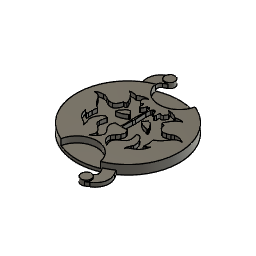
Deckbox - Key - Rakdos (Autodesk Fusion 360 design; units mm, degrees)
Autodesk Fusion 360 part; units mm, degrees
sketch "Sketch1" plane through (0, 0, 0) normal (0, 1, 0) x (1, 0, 0)
  circle A0 centre (0, 0) radius 25.4
  line L0 (19.5918, -28.934) -> (-15.2617, 31.434)
  line L1 (-19.5918, 28.934) -> (15.2617, -31.434)
  line L2 (0, -25.4) -> (0, 25.4) construction
  line L3 (0, 0) -> (25.4, 0) construction
  line L4 (-19.5918, 28.934) -> (-15.2617, 31.434)
  line L5 (15.2617, -31.434) -> (19.5918, -28.934)
  line L6 (17.4268, -30.184) -> (-17.4268, 30.184) construction
  line L7 (-2.1651, -1.25) -> (2.1651, 1.25) construction
  line L8 (19.5918, -28.934) -> (11.7976, -33.434)
  line L9 (11.7976, -33.434) -> (9.2976, -29.1039)
  line L10 (9.2976, -29.1039) -> (17.0918, -24.6039)
  line L11 (17.0918, -24.6039) -> (19.5918, -28.934)
  circle A1 centre (10.5476, -31.269) radius 2.5
  circle A2 centre (0, 0) radius 35.5
  line L12 (-19.5918, 28.934) -> (-17.0918, 24.6039)
  line L13 (-17.0918, 24.6039) -> (-9.2976, 29.1039)
  line L14 (-9.2976, 29.1039) -> (-11.7976, 33.434)
  line L15 (-11.7976, 33.434) -> (-19.5918, 28.934)
  circle A3 centre (-10.5476, 31.269) radius 2.5
  point P0 (-12.5, 21.6506)
  point P1 (12.5, -21.6506)
  dimension "d1" = 50.8
  dimension "d42" = 5
  dimension "d45" = 5
  dimension "d46" = 71
  dimension "d47" = 60
  dimension "d48" = 4
  dimension "d51" = 5
  constraint coincident A0.centre L3.start
  constraint coincident A0 L2.start
  constraint coincident A0 L2.end
  constraint coincident A0.centre L2
  constraint coincident A0 L3.end
  constraint horizontal L3
  constraint perpendicular L0 L4
  constraint perpendicular L0 L5
  constraint perpendicular L1 L4
  constraint midpoint L5 L6.start
  constraint midpoint L4 L6.end
  constraint perpendicular L4 L6
  constraint midpoint L1 L7.start
  constraint midpoint L0 L7.end
  constraint midpoint L6 A0.centre
  constraint perpendicular L8 L9
  constraint parallel L8 L10
  constraint parallel L9 L11
  constraint perpendicular L0 L8
  constraint midpoint L9 A1.centre
  constraint tangent L10 A1
  constraint concentric A0 A2
  constraint tangent A1 A2
  constraint perpendicular L12 L13
  constraint parallel L12 L14
  constraint parallel L13 L15
  constraint coincident L1 L12.end
  constraint midpoint L14 A3.centre
  constraint tangent L13 A3
  constraint tangent A2 A3
  measures "d1" diameter of A0
  measures "d42" distance of L0 L1
  measures "d45" diameter of A1
  measures "d46" diameter of A2 A0.centre
  measures "d47" angle of L3 L6
  measures "d48" distance of L1 A1.centre
  measures "d51" diameter of A3
extrude "Extrude1" add sketch "Sketch1" along normal blind 4.5 contours A0 L0 | A0 L0 L1 | A0 L1
extrude "Extrude2" add sketch "Sketch1" along normal blind 1.9 contours A0 L0 | A0 L0 L1 | A0 L0 L1 L13 | A0 L0 L1 L10 | A0 L1 | L0 L1 L4 L12 L13 L15 | L0 L13 L15 A3 | L0 L1 L5 L8 L10 L11 | L14 A3 | L14 A3 | L1 L8 L10 A1 | L9 A1 | L9 A1
extrude "Extrude3" add sketch "Sketch1" along normal blind 2.5 contours L14 A3 | L14 A3 | L9 A1 | L9 A1
sketch "Sketch2" plane through (0, 4.5, 0) normal (0, 1, 0) x (-1, 0, 0)
  circle A0 centre (0, 0) radius 25.4
  circle A1 centre (0, -25.4) radius 10
  circle A2 centre (0, 25.4) radius 10
  line L0 (0, -25.4) -> (0, 25.4) construction
  dimension "d18" = 20
  dimension "d19" = 20
  constraint coincident A0 A1.centre
  constraint coincident A0 A2.centre
  constraint coincident A1.centre L0.start
  constraint coincident A2.centre L0.end
  constraint coincident A0.centre L0
  constraint vertical L0
  measures "d18" diameter of A1
  measures "d19" diameter of A2
extrude "Extrude4" cut sketch "Sketch2" against normal blind 3 contours A0 A2 | A0 A1 picked at (-1.832, 22.0709) picked at (1.832, -22.0709)
fillet "Fillet6" radius 2 2 edges at (12.7617, 0.95, 27.1039) (-12.7617, 0.95, -27.1039)
fillet "Fillet7" radius 7 2 edges at (19.5918, 0.95, 28.934) (-19.5918, 0.95, -28.934)
sketch "Sketch3" plane through (0, 4.5, 0) normal (0, 1, 0) x (-1, 0, 0)
  arc A0 (-9.8043, 23.4315) -> (-9.8043, -23.4315) centre (0, 0) ccw
  spline S0 degree 3 poles (-4.3232, 14.8555) (-4.3232, 14.84) (-4.2479, 14.6896) (-4.114, 14.4374) knots 0 0 0 0 1 1 1 1
  spline S1 degree 3 poles (-4.114, 14.4374) (-3.4685, 13.2223) (-3.3365, 12.5312) (-3.5867, 11.6779) knots 0 0 0 0 1 1 1 1
  spline S2 degree 3 poles (-3.5867, 11.6779) (-3.8334, 10.8365) (-4.2867, 10.3197) (-5.7211, 9.2444) knots 0 0 0 0 1 1 1 1
  spline S3 degree 3 poles (-5.7211, 9.2444) (-6.746, 8.4761) (-7.0061, 8.2496) (-7.3329, 7.8412) knots 0 0 0 0 1 1 1 1
  spline S4 degree 3 poles (-7.3329, 7.8412) (-7.7451, 7.3262) (-7.9627, 6.6689) (-7.8957, 6.1401) knots 0 0 0 0 1 1 1 1
  spline S5 degree 3 poles (-7.8957, 6.1401) (-7.8192, 5.5352) (-7.453, 3.8698) (-7.2145, 3.0422) knots 0 0 0 0 1 1 1 1
  spline S6 degree 3 poles (-7.2145, 3.0422) (-7.1781, 2.9158) (-7.1519, 2.8094) (-7.1563, 2.8056) knots 0 0 0 0 1 1 1 1
  spline S7 degree 3 poles (-7.1563, 2.8056) (-7.1605, 2.8018) (-7.2159, 2.7934) (-7.2792, 2.7869) knots 0 0 0 0 1 1 1 1
  spline S8 degree 3 poles (-7.2792, 2.7869) (-7.4349, 2.771) (-7.9577, 2.711) (-8.2149, 2.6796) knots 0 0 0 0 1 1 1 1
  line L0 (-8.2149, 2.6796) -> (-8.424, 2.6541)
  line L1 (-8.424, 2.6541) -> (-8.5105, 2.7114)
  spline S9 degree 3 poles (-8.5105, 2.7114) (-9.2284, 3.1878) (-9.9979, 4.0729) (-10.5135, 5.0154) knots 0 0 0 0 1 1 1 1
  spline S10 degree 3 poles (-10.5135, 5.0154) (-11.1798, 6.2335) (-11.3977, 7.5273) (-11.0924, 8.4525) knots 0 0 0 0 1 1 1 1
  spline S11 degree 3 poles (-11.0924, 8.4525) (-11.0292, 8.6439) (-10.9777, 8.7574) (-10.7473, 9.2134) knots 0 0 0 0 1 1 1 1
  spline S12 degree 3 poles (-10.7473, 9.2134) (-10.4288, 9.844) (-10.3072, 10.1818) (-10.2108, 10.705) knots 0 0 0 0 1 1 1 1
  spline S13 degree 3 poles (-10.2108, 10.705) (-10.1491, 11.0402) (-10.0941, 11.5884) (-10.0956, 11.8545) knots 0 0 0 0 1 1 1 1
  line L2 (-10.0956, 11.8545) -> (-10.096, 11.9297)
  line L3 (-10.096, 11.9297) -> (-10.135, 11.8125)
  spline S14 degree 3 poles (-10.135, 11.8125) (-10.3374, 11.2033) (-10.7118, 10.8714) (-11.9958, 10.1624) knots 0 0 0 0 1 1 1 1
  spline S15 degree 3 poles (-11.9958, 10.1624) (-12.7961, 9.7205) (-13.1607, 9.495) (-13.5622, 9.1932) knots 0 0 0 0 1 1 1 1
  spline S16 degree 3 poles (-13.5622, 9.1932) (-14.8947, 8.1916) (-15.6884, 6.8114) (-16.0072, 4.9415) knots 0 0 0 0 1 1 1 1
  spline S17 degree 3 poles (-16.0072, 4.9415) (-16.0323, 4.794) (-16.0296, 4.7863) (-15.9839, 4.8766) knots 0 0 0 0 1 1 1 1
  spline S18 degree 3 poles (-15.9839, 4.8766) (-15.749, 5.3417) (-15.2485, 5.7388) (-14.8855, 5.7479) knots 0 0 0 0 1 1 1 1
  line L4 (-14.8855, 5.7479) -> (-14.7907, 5.7503)
  line L5 (-14.7907, 5.7503) -> (-14.7317, 5.8382)
  spline S19 degree 3 poles (-14.7317, 5.8382) (-14.4686, 6.2307) (-14.147, 6.5223) (-13.9762, 6.5233) knots 0 0 0 0 1 1 1 1
  spline S20 degree 3 poles (-13.9762, 6.5233) (-13.9206, 6.5236) (-13.9207, 6.5239) (-13.9435, 6.3922) knots 0 0 0 0 1 1 1 1
  spline S21 degree 3 poles (-13.9435, 6.3922) (-13.9836, 6.1605) (-14.019, 5.8212) (-14.0453, 5.4163) knots 0 0 0 0 1 1 1 1
  spline S22 degree 3 poles (-14.0453, 5.4163) (-14.0629, 5.1457) (-14.063, 3.8981) (-14.0455, 3.6225) knots 0 0 0 0 1 1 1 1
  spline S23 degree 3 poles (-14.0455, 3.6225) (-13.9774, 2.5472) (-13.8599, 1.834) (-13.6638, 1.3035) knots 0 0 0 0 1 1 1 1
  spline S24 degree 3 poles (-13.6638, 1.3035) (-13.6467, 1.2571) (-13.6336, 1.2182) (-13.635, 1.217) knots 0 0 0 0 1 1 1 1
  spline S25 degree 3 poles (-13.635, 1.217) (-13.6363, 1.2158) (-13.6892, 1.1889) (-13.7527, 1.1573) knots 0 0 0 0 1 1 1 1
  spline S26 degree 3 poles (-13.7527, 1.1573) (-14.5202, 0.7741) (-15.2509, 0.2522) (-15.8555, -0.3449) knots 0 0 0 0 1 1 1 1
  spline S27 degree 3 poles (-15.8555, -0.3449) (-16.4345, -0.9167) (-16.8065, -1.4006) (-17.5005, -2.4852) knots 0 0 0 0 1 1 1 1
  spline S28 degree 3 poles (-17.5005, -2.4852) (-18.1246, -3.4604) (-18.4276, -3.851) (-18.8281, -4.1974) knots 0 0 0 0 1 1 1 1
  spline S29 degree 3 poles (-18.8281, -4.1974) (-19.5229, -4.798) (-20.2555, -5.0448) (-21.5036, -5.0986) knots 0 0 0 0 1 1 1 1
  line L6 (-21.5036, -5.0986) -> (-21.664, -5.1056)
  line L7 (-21.664, -5.1056) -> (-21.6039, -5.1535)
  spline S30 degree 3 poles (-21.6039, -5.1535) (-21.2674, -5.4216) (-20.7454, -5.6937) (-20.2337, -5.8676) knots 0 0 0 0 1 1 1 1
  spline S31 degree 3 poles (-20.2337, -5.8676) (-19.1845, -6.2243) (-17.7553, -6.3205) (-16.9672, -6.0873) knots 0 0 0 0 1 1 1 1
  spline S32 degree 3 poles (-16.9672, -6.0873) (-16.6077, -5.9811) (-16.3618, -5.8552) (-15.8069, -5.4933) knots 0 0 0 0 1 1 1 1
  spline S33 degree 3 poles (-15.8069, -5.4933) (-15.0981, -5.0312) (-14.8175, -4.8913) (-14.3139, -4.7489) knots 0 0 0 0 1 1 1 1
  spline S34 degree 3 poles (-14.3139, -4.7489) (-13.6862, -4.5713) (-12.7854, -4.5135) (-12.307, -4.6201) knots 0 0 0 0 1 1 1 1
  spline S35 degree 3 poles (-12.307, -4.6201) (-11.2155, -4.8633) (-10.4225, -5.9028) (-9.9684, -7.6859) knots 0 0 0 0 1 1 1 1
  spline S36 degree 3 poles (-9.9684, -7.6859) (-9.9326, -7.8264) (-9.899, -7.9583) (-9.8937, -7.9789) knots 0 0 0 0 1 1 1 1
  line L8 (-9.8937, -7.9789) -> (-9.8839, -8.0165)
  line L9 (-9.8839, -8.0165) -> (-9.8344, -7.9914)
  spline S37 degree 3 poles (-9.8344, -7.9914) (-9.4661, -7.8047) (-9.0003, -7.8234) (-8.7851, -8.0334) knots 0 0 0 0 1 1 1 1
  spline S38 degree 3 poles (-8.7851, -8.0334) (-8.5675, -8.2459) (-8.6314, -8.5665) (-9.0766, -9.4946) knots 0 0 0 0 1 1 1 1
  spline S39 degree 3 poles (-9.0766, -9.4946) (-10.0976, -11.6236) (-11.5586, -13.2241) (-13.0137, -13.8076) knots 0 0 0 0 1 1 1 1
  spline S40 degree 3 poles (-13.0137, -13.8076) (-13.1416, -13.8589) (-13.1411, -13.8575) (-13.0478, -13.8967) knots 0 0 0 0 1 1 1 1
  spline S41 degree 3 poles (-13.0478, -13.8967) (-12.3642, -14.1837) (-10.9358, -14.1235) (-9.6156, -13.7521) knots 0 0 0 0 1 1 1 1
  line L10 (-9.6156, -13.7521) -> (-9.492, -13.7173)
  line L11 (-9.492, -13.7173) -> (-9.4096, -13.7964)
  spline S42 degree 3 poles (-9.4096, -13.7964) (-8.7246, -14.4541) (-7.3203, -15.0258) (-6.0462, -15.1659) knots 0 0 0 0 1 1 1 1
  spline S43 degree 3 poles (-6.0462, -15.1659) (-5.675, -15.2066) (-4.8009, -15.2092) (-4.9044, -15.1692) knots 0 0 0 0 1 1 1 1
  spline S44 degree 3 poles (-4.9044, -15.1692) (-4.9126, -15.1661) (-4.9487, -15.1535) (-4.9846, -15.1412) knots 0 0 0 0 1 1 1 1
  spline S45 degree 3 poles (-4.9846, -15.1412) (-5.6774, -14.9038) (-6.4552, -14.0325) (-6.46, -13.4885) knots 0 0 0 0 1 1 1 1
  spline S46 degree 3 poles (-6.46, -13.4885) (-6.4631, -13.1388) (-6.0298, -12.3937) (-5.5419, -11.9095) knots 0 0 0 0 1 1 1 1
  spline S47 degree 3 poles (-5.5419, -11.9095) (-4.927, -11.2995) (-4.4549, -11.3506) (-4.2518, -12.0497) knots 0 0 0 0 1 1 1 1
  spline S48 degree 3 poles (-4.2518, -12.0497) (-4.2241, -12.1449) (-4.2303, -12.1478) (-4.1399, -11.9973) knots 0 0 0 0 1 1 1 1
  spline S49 degree 3 poles (-4.1399, -11.9973) (-3.7726, -11.3854) (-3.7203, -10.8265) (-3.9765, -10.2475) knots 0 0 0 0 1 1 1 1
  line L12 (-3.9765, -10.2475) -> (-4.0011, -10.1919)
  line L13 (-4.0011, -10.1919) -> (-3.9349, -10.0737)
  spline S50 degree 3 poles (-3.9349, -10.0737) (-3.8628, -9.9448) (-3.7451, -9.7037) (-3.662, -9.5147) knots 0 0 0 0 1 1 1 1
  spline S51 degree 3 poles (-3.662, -9.5147) (-3.6329, -9.4485) (-3.603, -9.3823) (-3.5955, -9.3676) knots 0 0 0 0 1 1 1 1
  line L14 (-3.5955, -9.3676) -> (-3.5818, -9.3406)
  line L15 (-3.5818, -9.3406) -> (-3.5191, -9.3586)
  spline S52 degree 3 poles (-3.5191, -9.3586) (-2.8503, -9.5507) (-2.4025, -10.1704) (-2.0524, -11.3885) knots 0 0 0 0 1 1 1 1
  spline S53 degree 3 poles (-2.0524, -11.3885) (-1.9105, -11.882) (-1.9247, -11.86) (-1.8216, -11.7507) knots 0 0 0 0 1 1 1 1
  spline S54 degree 3 poles (-1.8216, -11.7507) (-1.5685, -11.4824) (-1.3668, -11.0199) (-1.4199, -10.8299) knots 0 0 0 0 1 1 1 1
  spline S55 degree 3 poles (-1.4199, -10.8299) (-1.4388, -10.7621) (-1.2673, -10.8106) (-1.1899, -10.895) knots 0 0 0 0 1 1 1 1
  spline S56 degree 3 poles (-1.1899, -10.895) (-1.0195, -11.0806) (-1.0394, -11.4423) (-1.2358, -11.7278) knots 0 0 0 0 1 1 1 1
  spline S57 degree 3 poles (-1.2358, -11.7278) (-1.2529, -11.7526) (-1.2669, -11.7771) (-1.2669, -11.7822) knots 0 0 0 0 1 1 1 1
  spline S58 degree 3 poles (-1.2669, -11.7822) (-1.2669, -11.8057) (-0.9842, -11.8254) (-0.8973, -11.8081) knots 0 0 0 0 1 1 1 1
  spline S59 degree 3 poles (-0.8973, -11.8081) (-0.8351, -11.7957) (-0.5203, -11.2526) (-0.3903, -10.9336) knots 0 0 0 0 1 1 1 1
  spline S60 degree 3 poles (-0.3903, -10.9336) (-0.1766, -10.4095) (-0.1031, -9.7731) (-0.1337, -8.7129) knots 0 0 0 0 1 1 1 1
  spline S61 degree 3 poles (-0.1337, -8.7129) (-0.1691, -7.4849) (-0.2863, -4.5446) (-0.3463, -3.3794) knots 0 0 0 0 1 1 1 1
  spline S62 degree 3 poles (-0.3463, -3.3794) (-0.36, -3.1128) (-0.3567, -3.0373) (-0.2798, -1.8739) knots 0 0 0 0 1 1 1 1
  spline S63 degree 3 poles (-0.2798, -1.8739) (-0.0416, 1.7283) (-0.0734, 3.2025) (-0.391, 3.2848) knots 0 0 0 0 1 1 1 1
  spline S64 degree 3 poles (-0.391, 3.2848) (-0.4793, 3.3077) (-2.0575, 3.264) (-2.811, 3.2178) knots 0 0 0 0 1 1 1 1
  spline S65 degree 3 poles (-2.811, 3.2178) (-2.8849, 3.2133) (-2.9468, 3.2107) (-2.9486, 3.2122) knots 0 0 0 0 1 1 1 1
  spline S66 degree 3 poles (-2.9486, 3.2122) (-3.0219, 3.2719) (-3.4405, 4.1501) (-3.5309, 4.4342) knots 0 0 0 0 1 1 1 1
  spline S67 degree 3 poles (-3.5309, 4.4342) (-3.7341, 5.072) (-3.6169, 5.9143) (-3.2156, 6.6989) knots 0 0 0 0 1 1 1 1
  spline S68 degree 3 poles (-3.2156, 6.6989) (-2.9879, 7.1442) (-2.7416, 7.4893) (-2.1247, 8.227) knots 0 0 0 0 1 1 1 1
  spline S69 degree 3 poles (-2.1247, 8.227) (-1.4476, 9.0368) (-1.2228, 9.3617) (-1.0473, 9.7841) knots 0 0 0 0 1 1 1 1
  spline S70 degree 3 poles (-1.0473, 9.7841) (-0.512, 11.0729) (-1.211, 12.5802) (-2.9954, 13.9853) knots 0 0 0 0 1 1 1 1
  spline S71 degree 3 poles (-2.9954, 13.9853) (-3.431, 14.3283) (-4.3232, 14.913) (-4.3232, 14.8555) knots 0 0 0 0 1 1 1 1
  spline S72 degree 3 poles (4.3948, 14.8337) (2.085, 13.4862) (0.8098, 11.7767) (1.0335, 10.3277) knots 0 0 0 0 1 1 1 1
  spline S73 degree 3 poles (1.0335, 10.3277) (1.1289, 9.7096) (1.3736, 9.294) (2.2851, 8.2019) knots 0 0 0 0 1 1 1 1
  spline S74 degree 3 poles (2.2851, 8.2019) (3.2602, 7.0337) (3.5961, 6.4199) (3.7281, 5.5658) knots 0 0 0 0 1 1 1 1
  spline S75 degree 3 poles (3.7281, 5.5658) (3.8181, 4.9834) (3.776, 4.6429) (3.5468, 4.1031) knots 0 0 0 0 1 1 1 1
  spline S76 degree 3 poles (3.5468, 4.1031) (3.4604, 3.8996) (3.1249, 3.2467) (3.0882, 3.2106) knots 0 0 0 0 1 1 1 1
  spline S77 degree 3 poles (3.0882, 3.2106) (3.0877, 3.21) (3.0267, 3.2133) (2.9528, 3.2178) knots 0 0 0 0 1 1 1 1
  spline S78 degree 3 poles (2.9528, 3.2178) (2.1966, 3.2641) (0.6228, 3.3076) (0.5314, 3.2847) knots 0 0 0 0 1 1 1 1
  spline S79 degree 3 poles (0.5314, 3.2847) (0.2599, 3.2166) (0.1948, 1.9885) (0.3319, -0.4759) knots 0 0 0 0 1 1 1 1
  spline S80 degree 3 poles (0.3319, -0.4759) (0.3512, -0.825) (0.3765, -1.2271) (0.4316, -2.0642) knots 0 0 0 0 1 1 1 1
  spline S81 degree 3 poles (0.4316, -2.0642) (0.4962, -3.0449) (0.5, -3.1334) (0.4873, -3.3591) knots 0 0 0 0 1 1 1 1
  spline S82 degree 3 poles (0.4873, -3.3591) (0.4473, -4.0807) (0.3505, -6.437) (0.2912, -8.1318) knots 0 0 0 0 1 1 1 1
  spline S83 degree 3 poles (0.2912, -8.1318) (0.2194, -10.192) (0.3076, -10.6895) (0.9177, -11.6626) knots 0 0 0 0 1 1 1 1
  spline S84 degree 3 poles (0.9177, -11.6626) (0.98, -11.7619) (1.0096, -11.8003) (1.0279, -11.8054) knots 0 0 0 0 1 1 1 1
  spline S85 degree 3 poles (1.0279, -11.8054) (1.0875, -11.8221) (1.3839, -11.8091) (1.407, -11.7889) knots 0 0 0 0 1 1 1 1
  spline S86 degree 3 poles (1.407, -11.7889) (1.4088, -11.7873) (1.3876, -11.7485) (1.36, -11.7025) knots 0 0 0 0 1 1 1 1
  spline S87 degree 3 poles (1.36, -11.7025) (1.1169, -11.2983) (1.1931, -10.8239) (1.5044, -10.8041) knots 0 0 0 0 1 1 1 1
  line L16 (1.5044, -10.8041) -> (1.568, -10.8)
  line L17 (1.568, -10.8) -> (1.5572, -10.8388)
  spline S88 degree 3 poles (1.5572, -10.8388) (1.5144, -10.9928) (1.6453, -11.3359) (1.859, -11.6293) knots 0 0 0 0 1 1 1 1
  spline S89 degree 3 poles (1.859, -11.6293) (1.9121, -11.7021) (2.0269, -11.8244) (2.0422, -11.8244) knots 0 0 0 0 1 1 1 1
  spline S90 degree 3 poles (2.0422, -11.8244) (2.0598, -11.8244) (2.0988, -11.7143) (2.1698, -11.4636) knots 0 0 0 0 1 1 1 1
  spline S91 degree 3 poles (2.1698, -11.4636) (2.4632, -10.4272) (2.7677, -9.8883) (3.2488, -9.5535) knots 0 0 0 0 1 1 1 1
  spline S92 degree 3 poles (3.2488, -9.5535) (3.3724, -9.4674) (3.601, -9.3643) (3.7062, -9.3471) knots 0 0 0 0 1 1 1 1
  spline S93 degree 3 poles (3.7062, -9.3471) (3.7205, -9.3448) (3.7426, -9.385) (3.8173, -9.5497) knots 0 0 0 0 1 1 1 1
  spline S94 degree 3 poles (3.8173, -9.5497) (3.9099, -9.7536) (4.0442, -10.0242) (4.1061, -10.1319) knots 0 0 0 0 1 1 1 1
  line L18 (4.1061, -10.1319) -> (4.1384, -10.188)
  line L19 (4.1384, -10.188) -> (4.0921, -10.3073)
  spline S95 degree 3 poles (4.0921, -10.3073) (3.8642, -10.8944) (3.9215, -11.4039) (4.2829, -12.0044) knots 0 0 0 0 1 1 1 1
  spline S96 degree 3 poles (4.2829, -12.0044) (4.3679, -12.1455) (4.3636, -12.1445) (4.3983, -12.0322) knots 0 0 0 0 1 1 1 1
  spline S97 degree 3 poles (4.3983, -12.0322) (4.5681, -11.4802) (4.9063, -11.3412) (5.3596, -11.6367) knots 0 0 0 0 1 1 1 1
  spline S98 degree 3 poles (5.3596, -11.6367) (5.9104, -11.9959) (6.5961, -13.0244) (6.5936, -13.4879) knots 0 0 0 0 1 1 1 1
  spline S99 degree 3 poles (6.5936, -13.4879) (6.5905, -14.0442) (5.8156, -14.909) (5.1063, -15.1477) knots 0 0 0 0 1 1 1 1
  line L20 (5.1063, -15.1477) -> (5.0211, -15.1763)
  line L21 (5.0211, -15.1763) -> (5.0963, -15.185)
  spline S100 degree 3 poles (5.0963, -15.185) (5.3371, -15.2126) (5.969, -15.1948) (6.3123, -15.1508) knots 0 0 0 0 1 1 1 1
  spline S101 degree 3 poles (6.3123, -15.1508) (7.5342, -14.994) (8.8905, -14.4277) (9.543, -13.8019) knots 0 0 0 0 1 1 1 1
  line L22 (9.543, -13.8019) -> (9.6306, -13.7178)
  line L23 (9.6306, -13.7178) -> (9.7559, -13.7527)
  spline S102 degree 3 poles (9.7559, -13.7527) (11.0479, -14.1129) (12.4459, -14.1816) (13.1279, -13.9183) knots 0 0 0 0 1 1 1 1
  spline S103 degree 3 poles (13.1279, -13.9183) (13.172, -13.9013) (13.2204, -13.8827) (13.2356, -13.8771) knots 0 0 0 0 1 1 1 1
  spline S104 degree 3 poles (13.2356, -13.8771) (13.2776, -13.8613) (13.2721, -13.8568) (13.1455, -13.8043) knots 0 0 0 0 1 1 1 1
  spline S105 degree 3 poles (13.1455, -13.8043) (11.7199, -13.212) (10.344, -11.7409) (9.3301, -9.725) knots 0 0 0 0 1 1 1 1
  spline S106 degree 3 poles (9.3301, -9.725) (8.9441, -8.9576) (8.7694, -8.4777) (8.8027, -8.2761) knots 0 0 0 0 1 1 1 1
  spline S107 degree 3 poles (8.8027, -8.2761) (8.8693, -7.873) (9.4545, -7.7317) (9.9778, -7.9926) knots 0 0 0 0 1 1 1 1
  line L24 (9.9778, -7.9926) -> (10.0243, -8.0157)
  line L25 (10.0243, -8.0157) -> (10.077, -7.8032)
  spline S108 degree 3 poles (10.077, -7.8032) (10.5426, -5.9241) (11.3276, -4.872) (12.4522, -4.6195) knots 0 0 0 0 1 1 1 1
  spline S109 degree 3 poles (12.4522, -4.6195) (12.974, -4.5023) (13.9512, -4.5823) (14.6092, -4.796) knots 0 0 0 0 1 1 1 1
  spline S110 degree 3 poles (14.6092, -4.796) (15.0391, -4.9356) (15.3073, -5.0754) (15.9437, -5.4913) knots 0 0 0 0 1 1 1 1
  spline S111 degree 3 poles (15.9437, -5.4913) (16.8766, -6.101) (17.276, -6.2253) (18.2518, -6.2097) knots 0 0 0 0 1 1 1 1
  spline S112 degree 3 poles (18.2518, -6.2097) (19.4387, -6.1906) (20.4639, -5.9359) (21.2947, -5.4533) knots 0 0 0 0 1 1 1 1
  spline S113 degree 3 poles (21.2947, -5.4533) (21.4746, -5.3489) (21.7754, -5.1436) (21.795, -5.1116) knots 0 0 0 0 1 1 1 1
  spline S114 degree 3 poles (21.795, -5.1116) (21.7977, -5.1075) (21.6771, -5.0987) (21.5272, -5.0921) knots 0 0 0 0 1 1 1 1
  spline S115 degree 3 poles (21.5272, -5.0921) (20.0614, -5.0271) (19.1818, -4.5976) (18.3665, -3.5492) knots 0 0 0 0 1 1 1 1
  spline S116 degree 3 poles (18.3665, -3.5492) (18.1795, -3.3085) (17.972, -3.0054) (17.6623, -2.5201) knots 0 0 0 0 1 1 1 1
  spline S117 degree 3 poles (17.6623, -2.5201) (16.4208, -0.575) (15.5104, 0.319) (13.9467, 1.1291) knots 0 0 0 0 1 1 1 1
  spline S118 degree 3 poles (13.9467, 1.1291) (13.8546, 1.1768) (13.7778, 1.2169) (13.7761, 1.2182) knots 0 0 0 0 1 1 1 1
  spline S119 degree 3 poles (13.7761, 1.2182) (13.7743, 1.2195) (13.7931, 1.2762) (13.8178, 1.3443) knots 0 0 0 0 1 1 1 1
  spline S120 degree 3 poles (13.8178, 1.3443) (13.9991, 1.8448) (14.1192, 2.5813) (14.1819, 3.5774) knots 0 0 0 0 1 1 1 1
  spline S121 degree 3 poles (14.1819, 3.5774) (14.2037, 3.9255) (14.2071, 5.0629) (14.1872, 5.3762) knots 0 0 0 0 1 1 1 1
  spline S122 degree 3 poles (14.1872, 5.3762) (14.1593, 5.8157) (14.1245, 6.1557) (14.0843, 6.3825) knots 0 0 0 0 1 1 1 1
  spline S123 degree 3 poles (14.0843, 6.3825) (14.059, 6.5252) (14.0597, 6.5272) (14.1297, 6.5215) knots 0 0 0 0 1 1 1 1
  spline S124 degree 3 poles (14.1297, 6.5215) (14.3059, 6.5068) (14.6184, 6.22) (14.8651, 5.8465) knots 0 0 0 0 1 1 1 1
  line L26 (14.8651, 5.8465) -> (14.9317, 5.7457)
  line L27 (14.9317, 5.7457) -> (14.9973, 5.7501)
  spline S125 degree 3 poles (14.9973, 5.7501) (15.3327, 5.772) (15.837, 5.3902) (16.1039, 4.9123) knots 0 0 0 0 1 1 1 1
  spline S126 degree 3 poles (16.1039, 4.9123) (16.1748, 4.7852) (16.1745, 4.785) (16.1445, 4.956) knots 0 0 0 0 1 1 1 1
  spline S127 degree 3 poles (16.1445, 4.956) (15.8139, 6.8367) (15.0337, 8.1929) (13.7108, 9.187) knots 0 0 0 0 1 1 1 1
  spline S128 degree 3 poles (13.7108, 9.187) (13.323, 9.4782) (12.9485, 9.7125) (12.2811, 10.081) knots 0 0 0 0 1 1 1 1
  spline S129 degree 3 poles (12.2811, 10.081) (11.3037, 10.6208) (11.0258, 10.8034) (10.7277, 11.1023) knots 0 0 0 0 1 1 1 1
  spline S130 degree 3 poles (10.7277, 11.1023) (10.4793, 11.3513) (10.3215, 11.609) (10.2562, 11.8721) knots 0 0 0 0 1 1 1 1
  spline S131 degree 3 poles (10.2562, 11.8721) (10.1817, 12.172) (10.2766, 11.0777) (10.3626, 10.6435) knots 0 0 0 0 1 1 1 1
  spline S132 degree 3 poles (10.3626, 10.6435) (10.468, 10.1121) (10.5952, 9.7706) (10.9231, 9.1389) knots 0 0 0 0 1 1 1 1
  spline S133 degree 3 poles (10.9231, 9.1389) (11.2794, 8.4528) (11.3632, 8.1483) (11.3632, 7.5406) knots 0 0 0 0 1 1 1 1
  spline S134 degree 3 poles (11.3632, 7.5406) (11.3633, 6.8311) (11.1981, 6.1524) (10.838, 5.3809) knots 0 0 0 0 1 1 1 1
  spline S135 degree 3 poles (10.838, 5.3809) (10.3415, 4.3174) (9.4405, 3.2211) (8.6354, 2.701) knots 0 0 0 0 1 1 1 1
  line L28 (8.6354, 2.701) -> (8.5621, 2.6536)
  line L29 (8.5621, 2.6536) -> (8.3949, 2.6746)
  spline S136 degree 3 poles (8.3949, 2.6746) (8.181, 2.7013) (7.5736, 2.771) (7.4127, 2.7872) knots 0 0 0 0 1 1 1 1
  line L30 (7.4127, 2.7872) -> (7.2891, 2.7996)
  line L31 (7.2891, 2.7996) -> (7.2936, 2.8253)
  spline S137 degree 3 poles (7.2936, 2.8253) (7.2961, 2.8393) (7.3237, 2.9389) (7.3551, 3.0463) knots 0 0 0 0 1 1 1 1
  spline S138 degree 3 poles (7.3551, 3.0463) (7.6304, 3.9914) (8.0284, 5.8619) (8.0399, 6.2647) knots 0 0 0 0 1 1 1 1
  spline S139 degree 3 poles (8.0399, 6.2647) (8.0602, 6.9772) (7.7303, 7.6602) (7.066, 8.2809) knots 0 0 0 0 1 1 1 1
  spline S140 degree 3 poles (7.066, 8.2809) (6.7857, 8.5428) (6.6073, 8.6855) (5.9105, 9.2059) knots 0 0 0 0 1 1 1 1
  spline S141 degree 3 poles (5.9105, 9.2059) (4.4664, 10.2841) (4.0069, 10.7957) (3.7439, 11.6191) knots 0 0 0 0 1 1 1 1
  spline S142 degree 3 poles (3.7439, 11.6191) (3.4743, 12.4624) (3.5977, 13.1949) (4.2018, 14.3388) knots 0 0 0 0 1 1 1 1
  spline S143 degree 3 poles (4.2018, 14.3388) (4.3378, 14.5964) (4.465, 14.8462) (4.465, 14.8556) knots 0 0 0 0 1 1 1 1
  spline S144 degree 3 poles (4.465, 14.8556) (4.465, 14.8672) (4.4374, 14.8585) (4.3948, 14.8337) knots 0 0 0 0 1 1 1 1
  spline S145 degree 3 poles (-7.4797, -1.9146) (-6.1342, -2.0194) (-4.7618, -2.5631) (-3.2241, -3.6002) knots 0 0 0 0 1 1 1 1
  line L32 (-3.2241, -3.6002) -> (-2.9417, -3.7907)
  line L33 (-2.9417, -3.7907) -> (-3.0196, -4.0172)
  spline S146 degree 3 poles (-3.0196, -4.0172) (-3.0624, -4.1418) (-3.1143, -4.3046) (-3.1349, -4.379) knots 0 0 0 0 1 1 1 1
  spline S147 degree 3 poles (-3.1349, -4.379) (-3.1933, -4.5897) (-3.1802, -4.5727) (-3.3397, -4.6435) knots 0 0 0 0 1 1 1 1
  spline S148 degree 3 poles (-3.3397, -4.6435) (-3.5916, -4.7551) (-3.6694, -4.841) (-3.8465, -5.2026) knots 0 0 0 0 1 1 1 1
  spline S149 degree 3 poles (-3.8465, -5.2026) (-4.135, -5.7917) (-4.2906, -5.8596) (-4.9193, -5.6706) knots 0 0 0 0 1 1 1 1
  spline S150 degree 3 poles (-4.9193, -5.6706) (-5.4087, -5.5234) (-5.8384, -5.2899) (-6.097, -5.0308) knots 0 0 0 0 1 1 1 1
  spline S151 degree 3 poles (-6.097, -5.0308) (-6.2119, -4.9156) (-6.2497, -4.861) (-6.4474, -4.5243) knots 0 0 0 0 1 1 1 1
  spline S152 degree 3 poles (-6.4474, -4.5243) (-6.8621, -3.8185) (-7.1861, -3.4354) (-7.5547, -3.215) knots 0 0 0 0 1 1 1 1
  spline S153 degree 3 poles (-7.5547, -3.215) (-7.6128, -3.1802) (-7.6162, -3.1727) (-7.5998, -3.1163) knots 0 0 0 0 1 1 1 1
  spline S154 degree 3 poles (-7.5998, -3.1163) (-7.5323, -2.885) (-7.5884, -2.6135) (-7.7756, -2.2646) knots 0 0 0 0 1 1 1 1
  spline S155 degree 3 poles (-7.7756, -2.2646) (-7.8125, -2.1957) (-7.8723, -2.0836) (-7.9083, -2.0152) knots 0 0 0 0 1 1 1 1
  line L34 (-7.9083, -2.0152) -> (-7.9738, -1.8912)
  line L35 (-7.9738, -1.8912) -> (-7.7895, -1.898)
  spline S156 degree 3 poles (-7.7895, -1.898) (-7.688, -1.9018) (-7.5486, -1.9092) (-7.4797, -1.9146) knots 0 0 0 0 1 1 1 1
  spline S157 degree 3 poles (8.0965, -1.9265) (8.0874, -1.9444) (8.0308, -2.0497) (7.9707, -2.1604) knots 0 0 0 0 1 1 1 1
  spline S158 degree 3 poles (7.9707, -2.1604) (7.7295, -2.605) (7.6727, -2.8313) (7.7353, -3.0997) knots 0 0 0 0 1 1 1 1
  spline S159 degree 3 poles (7.7353, -3.0997) (7.7452, -3.1428) (7.752, -3.1794) (7.7501, -3.1808) knots 0 0 0 0 1 1 1 1
  spline S160 degree 3 poles (7.7501, -3.1808) (7.7483, -3.1824) (7.7242, -3.1966) (7.6967, -3.2126) knots 0 0 0 0 1 1 1 1
  spline S161 degree 3 poles (7.6967, -3.2126) (7.3355, -3.4211) (7.01, -3.8064) (6.5845, -4.5293) knots 0 0 0 0 1 1 1 1
  spline S162 degree 3 poles (6.5845, -4.5293) (6.3604, -4.9103) (6.3046, -4.985) (6.1435, -5.1192) knots 0 0 0 0 1 1 1 1
  spline S163 degree 3 poles (6.1435, -5.1192) (5.8363, -5.3754) (5.306, -5.625) (4.8558, -5.7253) knots 0 0 0 0 1 1 1 1
  spline S164 degree 3 poles (4.8558, -5.7253) (4.3903, -5.8291) (4.2552, -5.7471) (3.9815, -5.1949) knots 0 0 0 0 1 1 1 1
  spline S165 degree 3 poles (3.9815, -5.1949) (3.804, -4.8367) (3.7261, -4.7518) (3.4724, -4.6404) knots 0 0 0 0 1 1 1 1
  spline S166 degree 3 poles (3.4724, -4.6404) (3.3322, -4.5788) (3.3286, -4.5748) (3.2926, -4.4391) knots 0 0 0 0 1 1 1 1
  spline S167 degree 3 poles (3.2926, -4.4391) (3.2757, -4.3758) (3.2275, -4.2225) (3.1854, -4.0985) knots 0 0 0 0 1 1 1 1
  spline S168 degree 3 poles (3.1854, -4.0985) (3.1434, -3.9744) (3.1032, -3.8539) (3.096, -3.8306) knots 0 0 0 0 1 1 1 1
  line L36 (3.096, -3.8306) -> (3.0832, -3.7881)
  line L37 (3.0832, -3.7881) -> (3.4259, -3.5595)
  spline S169 degree 3 poles (3.4259, -3.5595) (5.1019, -2.4416) (6.52, -1.928) (8.0201, -1.8958) knots 0 0 0 0 1 1 1 1
  line L38 (8.0201, -1.8958) -> (8.113, -1.8939)
  line L39 (8.113, -1.8939) -> (8.0965, -1.9265)
  arc A1 (-9.8043, 23.4315) -> (9.8043, 23.4315) centre (0, 25.4) ccw
  arc A2 (9.8043, -23.4315) -> (-9.8043, -23.4315) centre (0, -25.4) ccw
  arc A3 (9.8043, -23.4315) -> (9.8043, 23.4315) centre (0, 0) ccw
extrude "Extrude5" cut sketch "Sketch3" against normal blind 2 contours S0 S1 S2 S3 S4 S5 S6 S7 S8 L0 L1 S9 S10 S11 S12 S13 L2 L3 S14 S15 S16 S17 S18 L4 L5 S19 S20 S21 S22 S23 S24 S25 S26 S27 S28 S29 L6 L7 S30 S31 S32 S33 S34 S35 S36 L8 L9 S37 S38 S39 S40 S41 L10 L11 S42 S43 S44 S45 S46 S47 S48 S49 L12 L13 S50 S51 L14 L15 S52 S53 S54 S55 S56 S57 S58 S59 S60 S61 S62 S63 S64 S65 S66 S67 S68 S69 S70 S71 | S72 S73 S74 S75 S76 S77 S78 S79 S80 S81 S82 S83 S84 S85 S86 S87 L16 L17 S88 S89 S90 S91 S92 S93 S94 L18 L19 S95 S96 S97 S98 S99 L20 L21 S100 S101 L22 L23 S102 S103 S104 S105 S106 S107 L24 L25 S108 S109 S110 S111 S112 S113 S114 S115 S116 S117 S118 S119 S120 S121 S122 S123 S124 L26 L27 S125 S126 S127 S128 S129 S130 S131 S132 S133 S134 S135 L28 L29 S136 L30 L31 S137 S138 S139 S140 S141 S142 S143 S144
named bodies: "Deckbox - Key - Rakdos"
